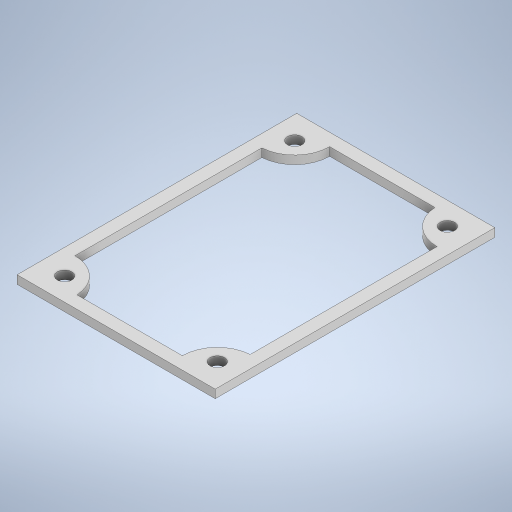
# Autodesk Inventor part: Pieza3
Saved by Autodesk Inventor 2024 (Build 280153000, 153)
## iProperties
Created: 2024-07-20
Part Number: Pieza3
Material: Genérico
Document SubType Name: Modeling
Designer: sergi
Density: 1 g/cm^3
Appearance: Valor por defecto
Author: sergi
Autodesk Inventor part; units mm, degrees
ref_plane "YZ Plane" through (0, 0, 0) normal (1, 0, 0) x (0, 1, 0)
ref_plane "XZ Plane" through (0, 0, 0) normal (0, 1, 0) x (-1, 0, 0)
ref_plane "XY Plane" through (0, 0, 0) normal (0, 0, 1) x (1, 0, 0)
sketch "Boceto1" plane through (0, 0, 0) normal (0, 1, 0) x (-1, 0, 0)
  line L0 (-23.8, -33.6) -> (23.8, -33.6)
  line L1 (23.8, -33.6) -> (23.8, 33.6)
  line L2 (23.8, 33.6) -> (-23.8, 33.6)
  line L3 (-23.8, 33.6) -> (-23.8, -33.6)
  line L4 (-12.4, -30.6) -> (12.9, -30.6)
  line L5 (12.4, 30.6) -> (-12.9, 30.6)
  line L6 (-23.8, 33.6) -> (-23.8, 29.4)
  circle A0 centre (-18.35, 27.65) radius 1.75
  line L7 (-16.6, 29.4) -> (-20.1, 25.9) construction
  line L8 (-20.1, 29.4) -> (-16.6, 25.9) construction
  line L9 (-12.9, 22.2) -> (-20.8, 22.2)
  line L10 (-23.8, 22.2) -> (-23.8, 33.1)
  line L11 (-12.9, 30.6) -> (-12.9, 22.2)
  line L12 (0, 33.6) -> (0, -33.6)
  line L13 (-23.8, 0) -> (23.8, 0)
  circle A1 centre (-17.85, -28.15) radius 1.75
  line L14 (-19.6, -26.4) -> (-16.1, -29.9) construction
  line L15 (-19.6, -29.9) -> (-16.1, -26.4) construction
  line L16 (-12.4, -22.7) -> (-12.4, -30.6)
  line L17 (-20.8, -22.7) -> (-12.4, -22.7)
  circle A2 centre (18.35, -27.65) radius 1.75
  line L18 (16.6, -29.4) -> (20.1, -25.9) construction
  line L19 (12.9, -22.2) -> (20.8, -22.2)
  line L20 (12.9, -30.6) -> (12.9, -22.2)
  circle A3 centre (17.85, 28.15) radius 1.75
  line L21 (19.6, 26.4) -> (16.1, 29.9) construction
  line L22 (19.6, 29.9) -> (16.1, 26.4) construction
  line L23 (12.4, 22.7) -> (12.4, 30.6)
  line L24 (20.8, 22.7) -> (12.4, 22.7)
  line L25 (20.8, -22.2) -> (20.8, 22.7)
  line L26 (-20.8, 22.2) -> (-20.8, -22.7)
  point P0 (0, 0)
  dimension "d0" = 47.6
  dimension "d1" = 67.2
  dimension "d3" = 4.2
  dimension "d5" = 3.5
  dimension "d9" = 3.5
  dimension "d11" = 3.5
  constraints: 54 end point, 11 midpoint, 5 parallel, 4 centre point, 2 perpendicular, 1 horizontal, 1 point on line
  measures "d0" distance of L2.end L1.end
  measures "d1" distance of L1.end L0.end
  measures "d3" distance of L2.end L6.end
  measures "d5" diameter of A0
  measures "d9" diameter of A2
  measures "d11" diameter of A3
extrude "Extrusión1" add sketch "Boceto1" along normal blind 2 contours L3 L13 L26 L17 L16 L4 L12 L0 | L12 L4 L20 L19 L25 L13 L1 L0 | L3 L2 L12 L5 L11 L9 L26 L13 | L13 L25 L24 L23 L5 L12 L2 L1
fillet "Empalme1" radius 8.4 4 edges at (-12.4, 1, 22.7) (12.9, 1, 22.2) (12.4, 1, -22.7) (-12.9, 1, -22.2)
